Autodesk Fusion 360 part; units mm, degrees
(part 4 of 4)
sketch "Boceto14" plane through (0, 0, 3) normal (0, 0, 1) x (-1, 0, 0)
  circle A0 centre (0, 0) radius 2
  circle A1 centre (-12.332883, -8.53815) radius 2
  circle A2 centre (12.332883, -8.53815) radius 2
  line L0 (43.868107, 21.148143) -> (-43.868107, 21.148143)
  line L1 (-43.868107, 21.148143) -> (-43.868107, -21.148143)
  line L2 (-43.868107, -21.148143) -> (43.868107, -21.148143)
  line L3 (43.868107, -21.148143) -> (43.868107, 21.148143)
  line L4 (-38.64619, 20.122863) -> (10, 20.122863)
  line L5 (10, 20.122863) -> (10, 7)
  line L6 (10, 7) -> (-38.64619, 7)
  line L7 (-38.64619, 7) -> (-38.64619, 20.122863)
  constraint horizontal L4
  constraint vertical L5
  constraint horizontal L6
  constraint vertical L7
extrude "Extruir4'" add sketch "Boceto14" along normal blind 25 contours L4 L5 L6 L7 picked at (-22.430793, 15.748575) bodies 24
sketch "Boceto15" plane through (0, 0, 28) normal (0, 0, 1) x (-1, 0, 0)
  line L0 (-38.64619, 7) -> (10, 7)
  line L1 (10, 7) -> (10, 20.122863)
  line L2 (10, 20.122863) -> (-38.64619, 20.122863)
  line L3 (-38.64619, 20.122863) -> (-38.64619, 7)
  line L4 (-28, -4) -> (-25, -4)
  line L5 (-25, -4) -> (-25, -8)
  line L6 (-25, -8) -> (-28, -8)
  line L7 (-28, -8) -> (-28, -4)
  constraint horizontal L4
  constraint vertical L5
  constraint horizontal L6
  constraint vertical L7
sketch "Boceto16" plane through (28, 0, 0) normal (1, 0, 0) x (0, 1, 0)
  line L0 (8, 28) -> (8, 34)
  line L1 (8, 34) -> (4, 34)
  line L2 (4, 34) -> (4, 28)
  circle A0 centre (6, 32) radius 1.414214
  line L3 (4, 28) -> (8, 28)
extrude "Extruir6'" cut sketch "Boceto16" against normal blind 5 contours A0 picked at (5.964772, 32.267032) bodies 24
sketch "Boceto17" plane through (0, 0, 28) normal (0, 0, 1) x (-1, 0, 0)
  line L0 (-38.64619, 7) -> (10, 7)
  line L1 (10, 7) -> (10, 20.122863)
  line L2 (10, 20.122863) -> (-38.64619, 20.122863)
  line L3 (-38.64619, 20.122863) -> (-38.64619, 7)
  line L4 (-10, 9) -> (-18, 9)
  line L5 (-18, 9) -> (-18, 12)
  line L6 (-18, 12) -> (-10, 12)
  line L7 (-10, 12) -> (-10, 9)
  line L8 (-10, 18.003846) -> (-18, 18.003846)
  line L9 (-18, 18.003846) -> (-18, 19.892521)
  line L10 (-18, 19.892521) -> (-10, 19.892521)
  line L11 (-10, 19.892521) -> (-10, 18.003846)
  constraint horizontal L4
  constraint vertical L5
  constraint horizontal L6
  constraint vertical L7
  constraint horizontal L8
  constraint vertical L9
  constraint horizontal L10
  constraint vertical L11
extrude "Extruir7" add sketch "Boceto17" along normal blind 9 contours L4 L5 L6 L7 picked at (-12.666667, 10) bodies 24
sketch "Boceto18" plane through (0, -12, 0) normal (0, -1, 0) x (1, 0, 0)
  line L0 (10, 28) -> (18, 28)
  line L1 (18, 28) -> (18, 37)
  line L2 (18, 37) -> (10, 37)
  line L3 (10, 37) -> (10, 28)
  circle A0 centre (14.323095, 32.284183) radius 2.691948
extrude "Extruir8" cut sketch "Boceto18" against normal blind 13 contours A0 picked at (14.522766, 31.488426) bodies 24
sketch "Boceto19" plane through (0, 0, 28) normal (0, 0, 1) x (-1, 0, 0)
  line L0 (-10, 12) -> (-10, 9)
  line L1 (-10, 9) -> (-18, 9)
  line L2 (-18, 9) -> (-18, 12)
  line L3 (-18, 12) -> (-10, 12)
  line L4 (-38.64619, 7) -> (10, 7)
  line L5 (10, 7) -> (10, 20.122863)
  line L6 (10, 20.122863) -> (-38.64619, 20.122863)
  line L7 (-38.64619, 20.122863) -> (-38.64619, 7)
extrude "Extruir9" add sketch "Boceto17" along normal blind 8 contours L8 L9 L10 L11 picked at (-12.666667, 18.633405) bodies 24
sketch "Boceto20" plane through (0, -19.892521, 0) normal (0, -1, 0) x (1, 0, 0)
  line L0 (10, 28) -> (18, 28)
  line L1 (18, 28) -> (18, 36)
  line L2 (18, 36) -> (10, 36)
  line L3 (10, 36) -> (10, 28)
  circle A0 centre (14.323095, 32.284183) radius 2.691948
  circle A1 centre (14.323095, 32.284183) radius 2.691948
  constraint concentric A0 A1
extrude "Extruir10" cut sketch "Boceto20" against normal blind 4 contours A0 A1 picked at (14.522766, 31.488426) bodies 24
sketch "Boceto1 (7)" plane through (0, 0, 0) normal (0, 0, 1) x (1, 0, 0) in component "Component'''"
  line L0 (1.875, 3.247595) -> (3.75, 0)
  line L1 (-1.875, 3.247595) -> (1.875, 3.247595)
  line L2 (-3.75, 0) -> (-1.875, 3.247595)
  line L3 (-1.875, -3.247595) -> (-3.75, 0)
  line L4 (1.875, -3.247595) -> (-1.875, -3.247595)
  line L5 (3.75, 0) -> (1.875, -3.247595)
extrude "Extruir1'''''''" add sketch "Boceto1 (7)" along normal blind 0.013 separate body contours L0 L1 L2 L3 L4 L5 picked at (0.625, -1.082532) makes body 28 in component "Component'''"
sketch "Boceto2 (7)" plane through (0, 0, 0) normal (0, 0, 1) x (1, 0, 0) in component "Component'''"
  circle A0 centre (0, 0) radius 2.5
extrude "Extruir2'''''''" add sketch "Boceto2 (7)" along normal blind 20 contours A0 picked at (-0.886301, 0.232065) bodies 28 in component "Component'''"
chamfer "Chaflán1''" distance 0.38 angle 45 1 edges at (-2.330818, -0.904039, 20) on bodies 28 in component "Component'''"
fillet "Empalme1''" radius 0.3 1 edges at (-2.330818, 0.904039, 0.013) on bodies 28 in component "Component'''"
sketch "Boceto3 (8)" plane through (0, 0, 0) normal (0, 1, 0) x (1, 0, 0) in component "Component'''"
  line L0 (3.247595, 0) -> (3.75, 0)
  line L1 (3.75, 0) -> (3.75, -0.290064)
  line L2 (3.75, -0.290064) -> (3.247595, 0)
sketch "Boceto4 (4)" plane through (0, 0, 0) normal (0, 1, 0) x (1, 0, 0) in component "Component'''"
  line L0 (3.247595, -0.013) -> (3.75, -0.013)
  line L1 (3.75, -0.013) -> (3.75, 0.277064)
  line L2 (3.75, 0.277064) -> (3.247595, -0.013)
revolve "Revolución1'''" cut sketch "Boceto4 (4)" angle 360 about axis through (0, 0, 1.75) along (0, 0, 1) contours L0 L1 L2 picked at (3.582532, 0.083688) bodies 28 in component "Component'''"
revolve "Revolución2''" cut sketch "Boceto3 (8)" angle 360 about axis through (0, 0, 1.75) along (0, 0, 1) contours L0 L1 L2 picked at (3.582532, -0.096688) bodies 28 in component "Component'''"
thread "Rosca1''" "ISO Metric profile 5.0 M5x0.8 6g" major diameter 4.901 minor diameter 3.9895 pitch 0.8 angle 60 resizes the face on face at (2.467626, 0.401028, 6.748667) on bodies 28 in component "Component'''"
extrude "Extruir4''" cut sketch "Boceto3 (7)" against normal blind 1.5 contours A1 picked at (3.031835, 19.661274) bodies 27 makes body 29 at (13.304725, 10.752391, 22) in component "Component''"
component "Spur Gear (20 teeth)" placed x (-0.9833578, -0.18167947, 0) y (-0.18167947, 0.9833578, 0) z (0, 0, -1) at (-12.332883, 8.53815, 4)
component "Spur Gear (20 teeth) (1)" placed x (-0.10014577, 0.99497278, 0) y (0.99497278, 0.10014577, 0) z (0, 0, -1) at (12.332883, 8.53815, 4)
component "Spur Gear (10 teeth)" placed x (0.33199322, -0.94328177, 0) y (-0.94328177, -0.33199322, 0) z (0, 0, -1) at (0, 0, 4)
component "Component" placed x (0.33933958, 0.94066394, 0) y (-0.94066394, 0.33933958, 0) z (0, 0, 1) at (40.905744, -7.377628, 4.231671)
component "Component'" placed x (0.33933958, 0.94066394, 0) y (-0.90861159, 0.32777686, -0.25881905) z (-0.24346174, 0.08782755, 0.96592583) at (15.545131, -16.293572, 13.65567)
component "Component''" placed x (-0.94066394, 0.33933958, 0) y (-0.33933958, -0.94066394, 0) z (0, 0, 1) at (24.36112, 13.261247, 0)
component "Component'''" placed x (-0.24694004, 0, 0.96903076) y (-0.96903076, 0, -0.24694004) z (0, -1, 0) at (14.323095, -6.366549, 32.284183)
equation "d262 = 360.0 * 10 deg"
named bodies: "Bolt"
